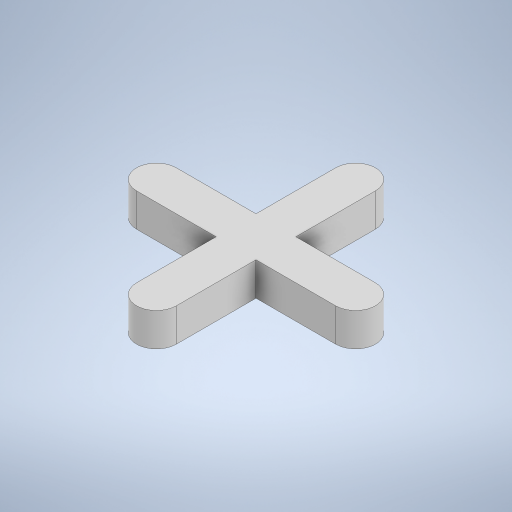
# Autodesk Inventor part: Part7 x 2
Saved by Autodesk Inventor 2023.1 (Build 271208000, 208)
## iProperties
Created: 2022-11-03
Part Number: Part7 x 2
Material: Generic
Document SubType Name: Modeling
Designer: jshin23
Density: 1 g/cm^3
Appearance: Default
Author: jshin23
Autodesk Inventor part; units mm, degrees
ref_plane "YZ Plane" through (0, 0, 0) normal (1, 0, 0) x (0, 1, 0)
ref_plane "XZ Plane" through (0, 0, 0) normal (0, 1, 0) x (-1, 0, 0)
ref_plane "XY Plane" through (0, 0, 0) normal (0, 0, 1) x (1, 0, 0)
sketch "Sketch1" plane through (0, 0, 0) normal (0, 1, 0) x (-1, 0, 0)
  line L0 (0, 0) -> (10.16, 0)
  line L1 (10.16, 0) -> (10.16, -5.08)
  line L2 (10.16, -5.08) -> (0, -5.08)
  line L3 (0, -5.08) -> (0, -15.24)
  line L4 (0, -15.24) -> (-5.08, -15.24)
  line L5 (-5.08, -15.24) -> (-5.08, -5.08)
  line L6 (-5.08, -5.08) -> (-15.24, -5.08)
  line L7 (-15.24, -5.08) -> (-15.24, 0)
  line L8 (-15.24, 0) -> (-5.08, 0)
  line L9 (-5.08, 0) -> (-5.08, 10.16)
  line L10 (-5.08, 10.16) -> (0, 10.16)
  line L11 (0, 10.16) -> (0, 0)
  arc A0 (10.16, -5.08) -> (10.16, 0) centre (10.16, -2.54) ccw
  arc A1 (-5.08, -15.24) -> (0, -15.24) centre (-2.54, -15.24) ccw
  arc A2 (-15.24, 0) -> (-15.24, -5.08) centre (-15.24, -2.54) ccw
  arc A3 (0, 10.16) -> (-5.08, 10.16) centre (-2.54, 10.16) ccw
  dimension "d0" = 10.16
  dimension "d1" = 5.08
  dimension "d2" = 10.16
  dimension "d3" = 5.08
  dimension "d4" = 10.16
  dimension "d5" = 10.16
  constraints: 24 end point, 8 perpendicular, 8 point on circle, 8 tangent, 7 point on line, 4 centre point, 1 horizontal
  measures "d0" distance of L0.start L0.end
  measures "d1" distance of L0.end L1.end
  measures "d2" distance of L2.end L3.end
  measures "d3" distance of L3.end L4.end
  measures "d4" distance of L5.end L6.end
  measures "d5" distance of L8.end L9.end
extrude "Extrusion1" add sketch "Sketch1" along normal blind 4.2418
body "Solid1"
